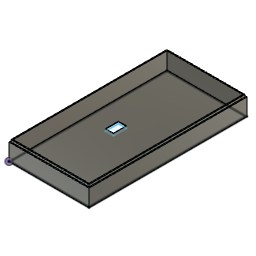
Case Parte de Baixo (Autodesk Fusion 360 design; units mm, degrees)
Autodesk Fusion 360 part; units mm, degrees
sketch "Sketch1" plane through (0, 0, 0) normal (0, 0, 1) x (1, 0, 0)
  line L0 (0, 0) -> (38, 0)
  line L1 (38, 0) -> (38, 75)
  line L2 (38, 75) -> (0, 75)
  line L3 (0, 75) -> (0, 0)
  line L4 (10.4482, 35.4042) -> (14.2003, 35.4042)
  line L5 (14.2003, 35.4042) -> (14.2003, 41.4905)
  line L6 (14.2003, 41.4905) -> (10.4482, 41.4905)
  line L7 (10.4482, 41.4905) -> (10.4482, 35.4042)
  line L8 (37.5, 0.5) -> (37.5, 74.5)
  line L9 (37.5, 74.5) -> (0.5, 74.5)
  line L10 (0.5, 74.5) -> (0.5, 0.5)
  line L11 (0.5, 0.5) -> (37.5, 0.5)
  dimension "d4" = 38
  dimension "d10" = -0.5
  dimension "d16" = 75
  constraint horizontal L0
  constraint vertical L1
  constraint horizontal L2
  constraint vertical L3
  constraint coincident L0.start L3.end
  constraint horizontal L4
  constraint vertical L5
  constraint horizontal L6
  constraint vertical L7
  measures "d4" distance of L1 L3
  measures "d16" distance of L0.start L2.end
extrude "Extrude1" add sketch "Sketch1" along normal blind 9 contours L0 L1 L2 L3 | L4 L5 L6 L7 | L8 L9 L10 L11
shell "Shell1" thickness 1 removed faces 1 at (12.6667, 50, 9)
extrude "Extrude2" cut sketch "Sketch1" along normal blind 1 contours L4 L5 L6 L7
extrude "Extrude3" cut sketch "Sketch1" against normal blind 1 from surface at 9 contours L0 L1 L2 L3
fillet "Fillet1" radius 0.75 4 edges at (12.3243, 35.4042, 0) (10.4482, 38.4474, 0) (14.2003, 38.4474, 0) (12.3243, 41.4905, 0)
